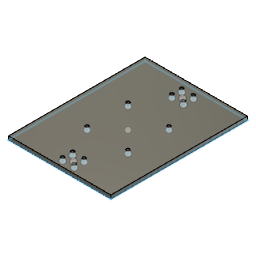
CNC Tartaro (Autodesk Fusion 360 design; units mm, degrees)
Autodesk Fusion 360 part; units mm, degrees
sketch "Boceto1" plane through (0, 0, 0) normal (0, 1, 0) x (1, 0, 0)
  line L0 (-25, 0) -> (125, 0)
  line L1 (125, 0) -> (125, 200)
  line L2 (125, 200) -> (-25, 200)
  line L3 (-25, 200) -> (-25, 0)
  circle A0 centre (20, 130) radius 2.5
  circle A1 centre (80, 130) radius 2.5
  circle A2 centre (20, 70) radius 2.5
  circle A3 centre (80, 70) radius 2.5
  circle A4 centre (41.5157, 172.7214) radius 2.5
  circle A5 centre (58.4843, 172.7214) radius 2.5
  circle A6 centre (41.5157, 187.2786) radius 2.5
  circle A7 centre (58.4843, 187.2786) radius 2.5
  circle A8 centre (41.5157, 27.2614) radius 2.5
  circle A9 centre (58.4843, 27.2614) radius 2.5
  circle A10 centre (41.5157, 12.7386) radius 2.5
  circle A11 centre (58.4843, 12.7386) radius 2.5
  point P0 (50, 100)
  point P1 (50, 180)
  point P2 (50, 20)
  dimension "d1" = 150
  dimension "d2" = 200
  dimension "d5" = 5
  dimension "d6" = 5
  dimension "d7" = 5
  dimension "d8" = 5
  dimension "d9" = 5
  dimension "d10" = 5
  dimension "d11" = 5
  dimension "d12" = 5
  dimension "d13" = 5
  dimension "d14" = 5
  dimension "d15" = 5
  dimension "d16" = 5
  constraint horizontal L0
  constraint vertical L1
  constraint horizontal L2
  constraint vertical L3
  measures "d1" distance of L0.start L0.end
  measures "d2" distance of L0.start L2.end
  measures "d5" diameter of A0
  measures "d6" diameter of A1
  measures "d7" diameter of A2
  measures "d8" diameter of A3
  measures "d9" diameter of A4
  measures "d10" diameter of A5
  measures "d11" diameter of A6
  measures "d12" diameter of A7
  measures "d13" diameter of A8
  measures "d14" diameter of A9
  measures "d15" diameter of A10
  measures "d16" diameter of A11
extrude "Extruir1" add sketch "Boceto1" along normal blind 1 contours L0 L1 L2 L3 | A0 | A1 | A2 | A3 | A4 | A5 | A6 | A7 | A8 | A9 | A10 | A11 makes body 1
extrude "Extruir2" add 1 faces at (25, 1, -133.3333) along direction (0, 1, 0) blind 4 on bodies 1 bodies 1
extrude "Extruir3" cut sketch "Boceto1" along normal blind 10 thin wall 1 on the right open curves A0 A2 A8 A10 A9 A11 A3 A1 A5 A7 A6 A4 bodies 1 makes body 2 at (42.3914, 1.6667, -173.9393) makes body 3 at (59.3599, 1.6667, -188.4965) makes body 4 at (80.4777, 1.6667, -131.4219) makes body 5 at (57.7999, 3.3333, -14.0734) makes body 6 at (40.8314, 3.3333, -14.0734) makes body 7 at (21.4095, 1.6667, -70.513) makes body 8 at (20.8756, 1.6667, -131.2179) makes body 9 at (40.8314, 3.3333, -28.5962) makes body 10 at (57.7999, 3.3333, -28.5962) makes body 11 at (81.4095, 1.6667, -70.513) makes body 12 at (59.3599, 1.6667, -173.9393) makes body 13 at (-10.8173, 5, -90.1626)
